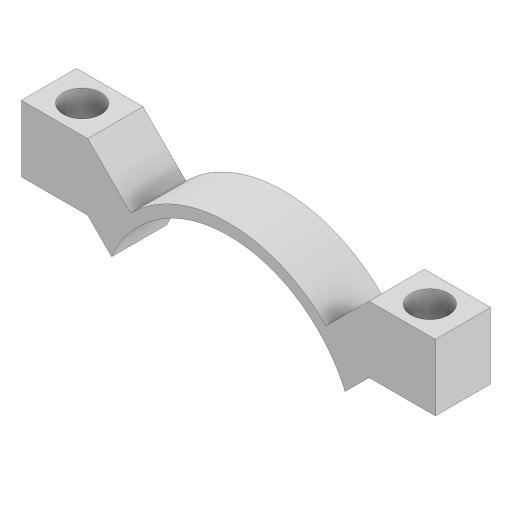
# Autodesk Inventor part: SOPORTE DE SENSOR INFRARROJO
Saved by Autodesk Inventor 2024 (Build 280153000, 153)
## iProperties
Created: 2024-07-05
Part Number: SOPORTE DE SENSOR INFRARROJO
Material: Generic
Document SubType Name: Modeling
Designer: Jhuliams
Density: 1 g/cm^3
Appearance: Default
Author: Jhuliams
Autodesk Inventor part; units mm, degrees
ref_plane "YZ Plane" through (0, 0, 0) normal (1, 0, 0) x (0, 1, 0)
ref_plane "XZ Plane" through (0, 0, 0) normal (0, 1, 0) x (-1, 0, 0)
ref_plane "XY Plane" through (0, 0, 0) normal (0, 0, 1) x (1, 0, 0)
sketch "Sketch3" plane through (0, 0, 0) normal (0, 0, 1) x (1, 0, 0)
  circle A0 centre (0, 0) radius 57.5
  line L0 (0, 0) -> (90, 0) construction
  line L1 (63.6396, 63.6396) -> (93.6396, 63.6396)
  line L2 (93.6396, 63.6396) -> (93.6396, 33.6396)
  line L3 (93.6396, 33.6396) -> (63.6396, 33.6396)
  line L4 (63.6396, 33.6396) -> (45, 15)
  line L5 (63.6396, 33.6396) -> (90, 33.6396) construction
  line L6 (-77.5, 7.5) -> (-47.5, 7.5)
  line L7 (-47.5, 7.5) -> (-47.5, -7.5)
  line L8 (-47.5, -7.5) -> (-77.5, -7.5)
  line L9 (-77.5, -7.5) -> (-77.5, 7.5)
  line L10 (-77.5, 7.5) -> (-47.5, -7.5) construction
  line L11 (-47.5, 7.5) -> (-77.5, -7.5) construction
  line L12 (0, 0) -> (40.6586, 40.6586)
  line L13 (44.1942, 44.1942) -> (63.6396, 63.6396)
  line L14 (0, 0) -> (0, 26.5707)
  line L15 (-63.6396, 63.6396) -> (-93.6396, 63.6396)
  line L16 (-93.6396, 63.6396) -> (-93.6396, 33.6396)
  line L17 (-93.6396, 33.6396) -> (-63.6396, 33.6396)
  line L18 (-63.6396, 33.6396) -> (-45, 15)
  line L19 (-63.6396, 33.6396) -> (-90, 33.6396) construction
  line L20 (-44.1942, 44.1942) -> (-63.6396, 63.6396)
  arc A1 (44.1942, 44.1942) -> (-44.1942, 44.1942) centre (0, 0) ccw
  arc A2 (-56.5707, 26.5707) -> (56.5707, 26.5707) centre (0, 0) ccw
  point P0 (-62.5, 0)
  point P1 (-57.0088, 7.5)
  point P2 (52.7905, 22.7905)
  point P3 (-40.6586, 40.6586)
  point P4 (-57.0088, -7.5)
  point P5 (-52.7905, 22.7905)
  dimension "d11" = 115
  dimension "d13" = 90
  dimension "d15" = 30
  dimension "d16" = 30
  dimension "d17" = 30
  dimension "d18" = 90
  dimension "d19" = 135
  dimension "d20" = 30
  dimension "d21" = 15
  constraints: 42 end point, 9 symmetric about line, 5 point on circle, 4 horizontal, 3 perpendicular, 2 centre point, 2 coincident, 2 midpoint, 2 parallel, 2 point on line, 1 equal length, 1 vertical, 3 other
  measures "d13" distance of L0.start L1.start
  measures "d15" distance of L1.start L1.end
  measures "d16" distance of L1.end L2.end
  measures "d17" distance of L2.end L3.end
  measures "d18" angle of L2 L3
  measures "d19" angle of L4 L5
  measures "d20" distance of L7.end L8.end
  measures "d21" distance of L6.end L7.end
extrude "Extrusion3" add sketch "Sketch3" against normal blind 25 contours A0 L18 L17 L16 L15 L20 A1 L13 L1 L2 L3 L4
sketch "Sketch6" plane through (63.6396, 63.6396, 0) normal (0, 1, 0) x (1, 0, 0)
  line L0 (30, 0) -> (0, 0) projected
  line L1 (30, 0) -> (30, 25) projected
  line L2 (0, 25) -> (30, 25) projected
  line L3 (0, 0) -> (0, 25) projected
  line L4 (30, 25) -> (0, 0)
  circle A0 centre (15, 12.5) radius 8.5
  point P0 (-63.6396, 0)
  dimension "d35" = 17
  constraints: 2 end point, 1 centre point, 1 midpoint
  measures "d35" diameter of A0
extrude "Extrusion6" cut sketch "Sketch6" against normal blind 40 contours A0 L4 | L4 A0
mirror "Mirror1" about plane through (0, 0, 0) normal (1, 0, 0) of "Extrusion6"
body "Solid2"
